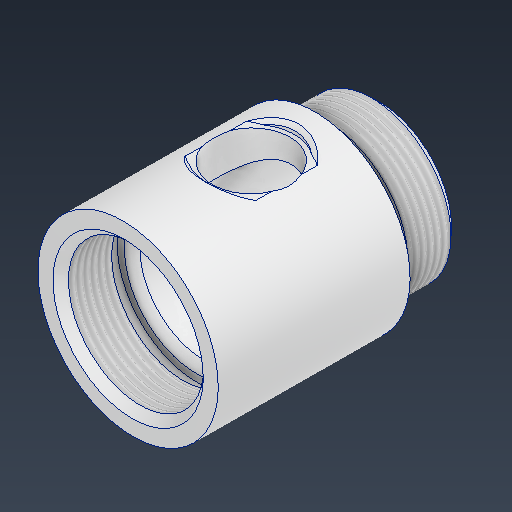
# Autodesk Inventor part: InventorNativeCentralControl
Saved by Autodesk Inventor 2025.1 (Build 291241000, 241)
## iProperties
Created: 2024-08-20
Part Number: InventorNativeCentralControl
Material: Aluminum 6061
Document SubType Name: Modeling
Designer: Michael
Density: 2.7 g/cm^3
Appearance: Aluminum - Flat
Mass: 64.2061 g
Surface Area: 113.839 cm^2
Volume: 23.78 cm^3
Author: Michael
Autodesk Inventor part; units mm, degrees
ref_plane "YZ Plane" through (0, 0, 0) normal (1, 0, 0) x (0, 1, 0)
ref_plane "XY Plane" through (0, 0, 0) normal (0, 0, 1) x (1, 0, 0)
sketch "Sketch1" plane through (0, 0, 0) normal (0, 0, 1) x (1, 0, 0)
  line L0 (-21.659, 0) -> (21.659, 0)
  line L1 (-15.24, 15.875) -> (-25.4, 15.875)
  line L2 (-25.4, 15.875) -> (-25.4, 12.7)
  line L3 (-25.4, 12.7) -> (12.7, 12.7)
  line L4 (12.7, 12.7) -> (12.7, 15.8115)
  line L5 (12.7, 15.8115) -> (15.24, 15.8115)
  line L6 (15.24, 15.8115) -> (15.24, 14.2875)
  line L7 (15.24, 14.2875) -> (25.4, 14.2875)
  line L8 (25.4, 14.2875) -> (25.4, 19.05)
  line L9 (25.4, 19.05) -> (-12.7, 19.05)
  line L10 (-12.7, 19.05) -> (-12.7, 15.113)
  line L11 (-12.7, 15.113) -> (-15.24, 15.113)
  line L12 (-15.24, 15.113) -> (-15.24, 15.875)
  line L13 (-25.4, 8.6409) -> (25.4, 8.6409) construction
  point P0 (0, 0)
  point P1 (0, 0)
  point P2 (0, 8.6409)
  dimension "d0" = 10.16
  dimension "d1" = 2.54
  dimension "d2" = 25.4
  dimension "d3" = 31.623
  dimension "d4" = 38.1
  dimension "d5" = 30.226
  dimension "d6" = 31.75
  dimension "d7" = 2.54
  dimension "d8" = 38.1
  dimension "d9" = 10.16
  dimension "d10" = 50.8
  dimension "d11" = 28.575
  constraints: 29 end point, 9 perpendicular, 3 horizontal, 3 vertical alignment, 2 midpoint, 1 coincident, 1 point on line, 1 vertical
  measures "d0" distance between parallel lines of L6 L8
  measures "d1" distance between parallel lines of L6 L4
  measures "d2" diameter of L3 L0
  measures "d3" diameter of L5 L0
  measures "d4" diameter of L9 L0
  measures "d5" diameter of L11 L0
  measures "d6" diameter of L1 L0
  measures "d7" distance between parallel lines of L10 L12
  measures "d8" distance between parallel lines of L8 L10
  measures "d9" distance between parallel lines of L2 L12
  measures "d10" distance of L13.start L13.end
  measures "d11" diameter of L7 L0
revolve "Revolution1" add sketch "Sketch1" angle 360 about axis through (-21.659, 0, 0) along (1, 0, 0)
thread "Thread1" size "1 1/8-18 UNEF" class "2B" standard "ANSI Unified Screw Threads" full length
thread "Thread2" size "1 1/4-18 UNEF" class "2A" standard "ANSI Unified Screw Threads" full length
chamfer "Chamfer1" distance 1.5875 angle 45 3 edges at (-25.4, -15.875, 0) (25.4, -14.2875, 0) (12.7, -12.7, 0)
ref_plane "Work Plane1" through (6.35, 19.05, 0) normal (0, 1, 0) x (-1, 0, 0)
sketch "Sketch2" plane through (6.35, 19.05, 0) normal (0, 1, 0) x (-1, 0, 0)
  line L0 (19.05, 19.05) -> (19.05, -19.05) projected
  line L1 (-19.05, 19.05) -> (-19.05, -19.05) projected
  circle A0 centre (5.6388, 0) radius 8
  point P0 (6.35, 0)
  point P1 (-2.3612, 0)
  point P2 (-19.05, 0)
  dimension "d21" = 16
  dimension "d22" = 24.6888
  constraints: 3 horizontal alignment, 1 midpoint, 2 other
  measures "d22" distance from line of L1 point (5.639, 0)
extrude "Extrusion1" cut sketch "Sketch2" against normal up to surface
sketch "Sketch3" plane through (6.35, 19.05, 0) normal (0, 1, 0) x (-1, 0, 0)
  circle A0 centre (5.6388, 0) radius 8
  line L0 (19.05, 0) -> (13.6388, 0) projected
  line L1 (-2.3612, 0) -> (-19.05, 0) projected
  circle A1 centre (5.6388, 0) radius 8.89
  point P0 (5.6388, -8)
  point P1 (13.4586, 0)
  point P2 (5.6388, 7.4676)
  dimension "d25" = 17.78
  constraints: 4 horizontal alignment, 2 centre point, 2 point on circle, 1 coincident, 1 vertical alignment, 3 other
  measures "d25" diameter of A1
extrude "Extrusion2" cut sketch "Sketch3" against normal blind 1.524
chamfer "Chamfer2" distance 0.7937 angle 45 4 edges at (8.3282, 18.4902, 4.5841) (-6.9058, 18.4902, 4.5841) (-6.9058, 18.4902, -4.5841) (8.3282, 18.4902, -4.5841)
body "Solid1"
